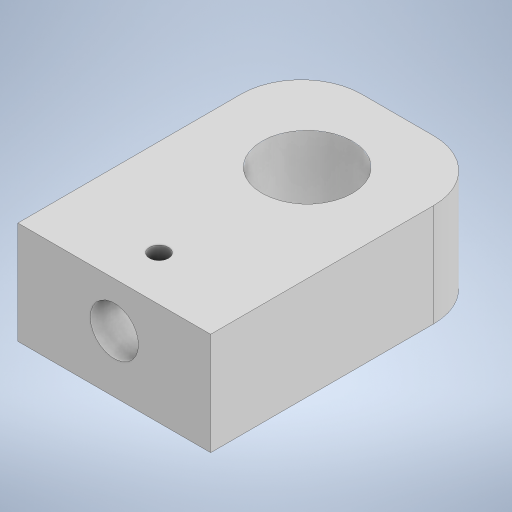
# Autodesk Inventor part: sujecion_v3
Saved by Autodesk Inventor 2023 (Build 270158000, 158)
## iProperties
Created: 2023-07-18
Part Number: sujecion_v3
Material: Generic
Document SubType Name: Modeling
Designer: checo
Density: 1 g/cm^3
Appearance: Default
Author: checo
Autodesk Inventor part; units mm, degrees
ref_plane "YZ Plane" through (0, 0, 0) normal (1, 0, 0) x (0, 1, 0)
ref_plane "XZ Plane" through (0, 0, 0) normal (0, 1, 0) x (-1, 0, 0)
ref_plane "XY Plane" through (0, 0, 0) normal (0, 0, 1) x (1, 0, 0)
sketch "Sketch1" plane through (0, 0, 0) normal (0, 0, 1) x (1, 0, 0)
  circle A0 centre (0, 0) radius 7.5
  line L0 (-16, 7.5) -> (16, 7.5)
  line L1 (16, 7.5) -> (16, -9.5)
  line L2 (16, -9.5) -> (-16, -9.5)
  line L3 (-16, -9.5) -> (-16, 7.5)
  line L4 (-7.5, 0) -> (-7.5, 7.5)
  line L5 (7.5, 0) -> (7.5, 7.5)
  point P0 (0, -9.5)
  dimension "d0" = 15
  dimension "d5" = 32
  dimension "d6" = 2
  constraints: 13 end point, 3 perpendicular, 3 tangent, 2 point on circle, 2 point on line, 1 centre point, 1 coincident, 1 horizontal, 1 midpoint, 1 parallel, 1 vertical, 1 vertical alignment
  measures "d0" diameter of A0
  measures "d5" distance of L1.end L2.end
  measures "d6" distance edge to line of A0 L2
extrude "Extrusion1" add sketch "Sketch1" along normal blind 24.2 contours A0 L5 L0 L1 L2 L3 L4
sketch "Sketch2" plane through (0, 0, 24.2) normal (0, 0, 1) x (1, 0, 0)
  line L0 (-16, -9.5) -> (16, -9.5) projected
  line L1 (16, -9.5) -> (16, 7.5) projected
  line L2 (16, 7.5) -> (7.5, 7.5) projected
  line L3 (7.5, 7.5) -> (7.5, 0) projected
  arc A0 (-7.5, 0) -> (7.5, 0) centre (0, 0) ccw projected
  line L4 (-7.5, 0) -> (-7.5, 7.5) projected
  line L5 (-7.5, 7.5) -> (-16, 7.5) projected
  line L6 (-16, 7.5) -> (-16, -9.5) projected
  circle A1 centre (0, 0) radius 4.25
  line L7 (-7.5, 7.5) -> (-16, 7.5) projected
  line L8 (-7.5, 7.5) -> (7.5, 7.5)
  dimension "d10" = 8.5
  constraints: 2 end point, 1 centre point, 1 coincident, 1 collinear
  measures "d10" diameter of A1
extrude "Extrusion3" add sketch "Sketch2" along normal blind 3
sketch "Sketch4" plane through (0, 0, 0) normal (0, 0, -1) x (-1, 0, 0)
  line L0 (-16, 7.5) -> (-7.5, 7.5) projected
  line L1 (-16, -9.5) -> (-16, 7.5) projected
  line L2 (16, -9.5) -> (-16, -9.5) projected
  line L3 (16, 7.5) -> (16, -9.5) projected
  line L4 (7.5, 7.5) -> (16, 7.5) projected
  line L5 (-7.5, 7.5) -> (7.5, 7.5) projected
  circle A0 centre (0, 0) radius 4.25 projected
extrude "Extrusion4" add sketch "Sketch4" along normal blind 3
sketch "Sketch5" plane through (0, 0, -3) normal (0, 0, -1) x (-1, 0, 0)
  line L0 (16, 7.5) -> (-16, 7.5) projected
  line L1 (16, -9.5) -> (16, 7.5) projected
  line L2 (-16, -9.5) -> (16, -9.5) projected
  line L3 (-16, 7.5) -> (-16, -9.5) projected
  circle A0 centre (0, 0) radius 7.5
  arc A1 (-7.5, 0) -> (7.5, 0) centre (0, 0) ccw projected
  line L4 (7.5, 0) -> (7.5, 7.5)
  line L5 (-16, 7.5) -> (16, 7.5) projected
  line L6 (-7.5, 7.5) -> (-7.5, 0) projected
  line L7 (-7.5, 0) -> (-7.5, 7.5)
  constraints: 4 end point, 3 tangent, 1 centre point, 1 coincident, 1 collinear, 1 perpendicular, 1 point on line
extrude "Extrusion5" add sketch "Sketch5" along normal blind 130 contours L1 L2 L3 L0 L6 A0 L4
sketch "Sketch6" plane through (0, 0, -133) normal (0, 0, -1) x (-1, 0, 0)
  line L0 (0, 0) -> (0, -9.5) construction
  line L1 (16, -9.5) -> (-16, -9.5) construction
  line L2 (-16, 7.5) -> (-16, -9.5) construction
  point P0 (-12.5, -6)
  point P1 (12.5, -6)
  dimension "d17" = 3.5
  dimension "d18" = 3.5
  constraints: 2 end point, 1 midpoint, 1 symmetric about line
  measures "d17" distance from line of point (-12.5, -6) L2
  measures "d18" distance from line of L1 point (-12.5, -6)
hole "Hole1" at (12.5, -6, -133) at (-12.5, -6, -133) direction (0, 0, 1) diameter 2.3813 depth 10 tip angle 118
sketch "Sketch7" plane through (-16, 7.5, 27.2) normal (0, 1, 0) x (1, 0, 0)
  line L0 (16, 0) -> (16, 160.2) construction
  line L1 (32, 160.2) -> (0, 160.2) projected
  line L2 (0, 160.2) -> (0, 0) projected
  line L3 (32, 0) -> (0, 0) projected
  point P0 (16, 27.2)
  point P1 (3.5, 3.5)
  point P2 (3.5, 33.5)
  point P3 (3.5, 63.5)
  point P4 (3.5, 93.5)
  point P5 (3.5, 123.5)
  point P6 (3.5, 145.2)
  point P7 (28.5, 3.5)
  point P8 (28.5, 33.5)
  point P9 (28.5, 63.5)
  point P10 (28.5, 93.5)
  point P11 (28.5, 123.5)
  point P12 (28.5, 145.2)
  dimension "d27" = 3.5
  dimension "d44" = 30
  dimension "d49" = 3.5
  dimension "d50" = 15
  constraints: 6 symmetric about line, 2 end point, 2 midpoint, 1 vertical, 1 vertical alignment, 4 other
  measures "d27" distance from line of L2 point (3.5, 3.5)
  measures "d44" distance of point (3.5, 3.5) point (3.5, 33.5)
  measures "d49" distance from line of L3 point (3.5, 3.5)
  measures "d50" distance from line of L1 point (3.5, 145.2)
hole "Hole3" at (-12.5, 7.5, 23.7) at (-12.5, 7.5, -6.3) at (-12.5, 7.5, -36.3) at (-12.5, 7.5, -66.3) at (-12.5, 7.5, -96.3) at (-12.5, 7.5, -118) at (12.5, 7.5, 23.7) at (12.5, 7.5, -6.3) at (12.5, 7.5, -36.3) at (12.5, 7.5, -66.3) at (12.5, 7.5, -96.3) at (12.5, 7.5, -118) direction (0, -1, 0) diameter 3.175 end through all
sketch "Sketch8" plane through (-16, -9.5, 27.2) normal (0, -1, 0) x (1, 0, 0)
  circle A0 centre (28.5, -3.5) radius 1.5875 projected
  line L0 (30.2321, -6.5) -> (26.7679, -6.5)
  line L1 (26.7679, -6.5) -> (25.0359, -3.5)
  line L2 (25.0359, -3.5) -> (26.7679, -0.5)
  line L3 (26.7679, -0.5) -> (30.2321, -0.5)
  line L4 (30.2321, -0.5) -> (31.9641, -3.5)
  line L5 (31.9641, -3.5) -> (30.2321, -6.5)
  line L6 (5.2321, -6.5) -> (1.7679, -6.5)
  line L7 (1.7679, -0.5) -> (5.2321, -0.5)
  line L8 (5.2321, -0.5) -> (6.9641, -3.5)
  line L9 (6.9641, -3.5) -> (5.2321, -6.5)
  line L10 (1.7679, -6.5) -> (0.0359, -3.5)
  line L11 (0.0359, -3.5) -> (1.7679, -0.5)
  line L12 (0, 0) -> (0, -160.2) projected
  line L13 (1.7679, -36.5) -> (0.0359, -33.5)
  line L14 (0.0359, -33.5) -> (1.7679, -30.5)
  line L15 (1.7679, -30.5) -> (5.2321, -30.5)
  line L16 (5.2321, -30.5) -> (6.9641, -33.5)
  line L17 (6.9641, -33.5) -> (5.2321, -36.5)
  line L18 (25.0359, -33.5) -> (26.7679, -30.5)
  line L19 (26.7679, -36.5) -> (25.0359, -33.5)
  line L20 (30.2321, -36.5) -> (26.7679, -36.5)
  line L21 (31.9641, -33.5) -> (30.2321, -36.5)
  line L22 (30.2321, -30.5) -> (31.9641, -33.5)
  line L23 (26.7679, -30.5) -> (30.2321, -30.5)
  line L24 (1.7679, -66.5) -> (0.0359, -63.5)
  line L25 (0.0359, -63.5) -> (1.7679, -60.5)
  line L26 (1.7679, -60.5) -> (5.2321, -60.5)
  line L27 (5.2321, -60.5) -> (6.9641, -63.5)
  line L28 (6.9641, -63.5) -> (5.2321, -66.5)
  line L29 (25.0359, -63.5) -> (26.7679, -60.5)
  line L30 (26.7679, -66.5) -> (25.0359, -63.5)
  line L31 (30.2321, -66.5) -> (26.7679, -66.5)
  line L32 (31.9641, -63.5) -> (30.2321, -66.5)
  line L33 (30.2321, -60.5) -> (31.9641, -63.5)
  line L34 (26.7679, -60.5) -> (30.2321, -60.5)
  line L35 (1.7679, -96.5) -> (0.0359, -93.5)
  line L36 (0.0359, -93.5) -> (1.7679, -90.5)
  line L37 (1.7679, -90.5) -> (5.2321, -90.5)
  line L38 (5.2321, -90.5) -> (6.9641, -93.5)
  line L39 (6.9641, -93.5) -> (5.2321, -96.5)
  line L40 (25.0359, -93.5) -> (26.7679, -90.5)
  line L41 (26.7679, -96.5) -> (25.0359, -93.5)
  line L42 (30.2321, -96.5) -> (26.7679, -96.5)
  line L43 (31.9641, -93.5) -> (30.2321, -96.5)
  line L44 (30.2321, -90.5) -> (31.9641, -93.5)
  line L45 (26.7679, -90.5) -> (30.2321, -90.5)
  line L46 (1.7679, -126.5) -> (0.0359, -123.5)
  line L47 (0.0359, -123.5) -> (1.7679, -120.5)
  line L48 (1.7679, -120.5) -> (5.2321, -120.5)
  line L49 (5.2321, -120.5) -> (6.9641, -123.5)
  line L50 (6.9641, -123.5) -> (5.2321, -126.5)
  line L51 (25.0359, -123.5) -> (26.7679, -120.5)
  line L52 (26.7679, -126.5) -> (25.0359, -123.5)
  line L53 (30.2321, -126.5) -> (26.7679, -126.5)
  line L54 (31.9641, -123.5) -> (30.2321, -126.5)
  line L55 (30.2321, -120.5) -> (31.9641, -123.5)
  line L56 (26.7679, -120.5) -> (30.2321, -120.5)
  line L57 (5.2321, -36.5) -> (1.7679, -36.5)
  line L58 (5.2321, -66.5) -> (1.7679, -66.5)
  line L59 (5.2321, -96.5) -> (1.7679, -96.5)
  line L60 (5.2321, -126.5) -> (1.7679, -126.5)
  line L61 (30.2321, -148) -> (26.7679, -148)
  line L62 (31.9641, -145) -> (30.2321, -148)
  line L63 (30.2321, -142) -> (31.9641, -145)
  line L64 (26.7679, -142) -> (30.2321, -142)
  line L65 (25.0359, -145) -> (26.7679, -142)
  line L66 (26.7679, -148) -> (25.0359, -145)
  line L67 (5.2321, -142) -> (6.9641, -145)
  line L68 (6.9641, -145) -> (5.2321, -148)
  line L69 (5.2321, -148) -> (1.7679, -148)
  line L70 (1.7679, -148) -> (0.0359, -145)
  line L71 (0.0359, -145) -> (1.7679, -142)
  line L72 (1.7679, -142) -> (5.2321, -142)
  point P0 (16, -27.2)
  point P1 (1.7679, -126.5)
  point P2 (5.2321, -126.5)
  dimension "d58" = 6
  dimension "d61" = 25
  dimension "d68" = 30
  dimension "d75" = 30
  dimension "d82" = 21.5
  constraints: 144 end point, 3 vertical, 2 horizontal, 1 coincident, 1 collinear, 154 other
  measures "d58" distance between parallel lines of L3 L0
  measures "d61" distance of L0.start L6.start
  measures "d68" distance of L6.end L13.start
  measures "d75" distance of L6.start L57.start
  measures "d82" distance of L53.start L61.start
extrude "Extrusion6" cut sketch "Sketch8" against normal blind 4 contours A0 | L0 L1 L2 L3 L4 L5 | L6 L10 L11 L7 L8 L9 | L13 L14 L15 L16 L17 L57 | L18 L23 L22 L21 L20 L19 | L24 L25 L26 L27 L28 L58 | L29 L34 L33 L32 L31 L30 | L35 L36 L37 L38 L39 L59 | L40 L45 L44 L43 L42 L41 | L46 L47 L48 L49 L50 L60 | L51 L56 L55 L54 L53 L52 | L61 L66 L65 L64 L63 L62 | L67 L68 L69 L70 L71 L72
sketch "Sketch9" plane through (0, 0, -133) normal (0, 0, -1) x (-1, 0, 0)
  line L0 (-15.9641, -9.5) -> (-15.9641, -5.5) projected
  line L1 (16, 7.5) -> (16, -9.5) projected
  line L2 (-15.9641, -9.5) -> (16, -9.5)
  line L3 (16, -9.5) -> (16, 7.5)
  line L4 (16, 7.5) -> (-15.9641, 7.5)
  line L5 (-15.9641, 7.5) -> (-15.9641, -9.5)
  point P0 (0, 0)
  constraints: 8 end point, 2 parallel, 1 horizontal, 1 perpendicular
extrude "Extrusion7" add sketch "Sketch9" along normal blind 50
fillet "Fillet1" radius 10 2 edges at (15.9641, -1, -183) (-16, -1, -183)
sketch "Sketch10" plane through (-16, 7.5, 27.2) normal (0, 1, 0) x (1, 0, 0)
  line L0 (10, 210.2) -> (21.9641, 210.2) projected
  point P0 (16, 27.2)
  point P1 (15.9821, 195.2)
  point P2 (15.9821, 210.2)
  point P3 (15.9821, 210.2)
  dimension "d94" = 15
  constraints: 2 midpoint, 1 vertical alignment
  measures "d94" distance of point (15.982, 210.2) point (15.982, 195.2)
hole "Hole4" at (-0.0179, 7.5, -168) direction (0, -1, 0) diameter 15 end through all
sketch "Sketch11" plane through (-16, 7.5, 27.2) normal (0, 1, 0) x (1, 0, 0)
  line L0 (28.5, 160.2) -> (3.5, 160.2)
  line L1 (3.5, 160.2) -> (3.5, 163.2)
  line L2 (3.5, 163.2) -> (28.5, 163.2)
  line L3 (28.5, 163.2) -> (28.5, 160.2)
  line L4 (8.5, 160.2) -> (23.5, 160.2) projected
  point P0 (16, 27.2)
  point P1 (3.5, 161.7)
  point P2 (16, 160.2)
  dimension "d102" = 25
  dimension "d103" = 3
  constraints: 8 end point, 3 midpoint, 2 parallel, 1 collinear, 1 horizontal, 1 perpendicular
  measures "d102" distance from line of point (3.5, 161.7) L3
  measures "d103" distance between parallel lines of L2 L0
extrude "Extrusion8" cut sketch "Sketch11" against normal blind 15
sketch "Sketch12" plane through (-12.5, 7.5, -136) normal (0, 0, 1) x (1, 0, 0)
  line L0 (-20.042, -34.0875) -> (45.042, -34.0875)
  line L1 (45.042, -34.0875) -> (45.042, 19.0875)
  line L2 (45.042, 19.0875) -> (-20.042, 19.0875)
  line L3 (-20.042, 19.0875) -> (-20.042, -34.0875)
  line L4 (-20.042, -34.0875) -> (45.042, 19.0875) construction
  line L5 (45.042, -34.0875) -> (-20.042, 19.0875) construction
  point P0 (12.5, -7.5)
  constraints: 12 end point, 2 midpoint, 2 parallel, 1 horizontal, 1 perpendicular
extrude "Extrusion9" cut sketch "Sketch12" along normal through all
sketch "Sketch13" plane through (-16, 7.5, -136) normal (0, 0, 1) x (1, 0, 0)
  circle A0 centre (16, -7.5) radius 4
  dimension "d108" = 8
  constraints: 1 centre point, 1 coincident
  measures "d108" diameter of A0
extrude "Extrusion10" cut sketch "Sketch13" against normal blind 10
sketch "Sketch14" plane through (-6, 7.5, -183) normal (0, 1, 0) x (1, 0, 0)
  circle A0 centre (5.9821, -39.5797) radius 1.5875
  point P0 (6, -183)
  dimension "d111" = 3.175
  constraints: 1 centre point
  measures "d111" diameter of A0
extrude "Extrusion11" cut sketch "Sketch14" against normal blind 10
body "Solid1"
